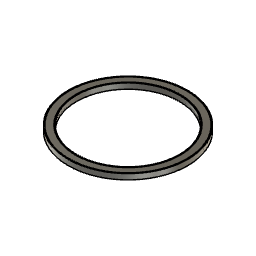
silicon_gasket_mold (Autodesk Fusion 360 design; units mm, degrees)
Autodesk Fusion 360 part; units mm, degrees
sketch "Sketch1" plane through (0, 0, 0) normal (0, 0, 1) x (1, 0, 0)
  circle A0 centre (0, 0) radius 91.5
  circle A1 centre (0, 0) radius 93
  circle A2 centre (0, 0) radius 81.5
  circle A3 centre (0, 0) radius 80
  line L0 (0, 0) -> (-81.5, 0) construction
  line L1 (-91.5, 0, 0) -> (-91.5, 0, 2.6785)
  line L2 (-81.5, 0, 0) -> (-91.5, 0, 2.6785)
  line L3 (-91.5, 0) -> (-81.5, 0)
  dimension "d1" = 183
  dimension "d2" = 1.5
  dimension "d3" = 163
  dimension "d4" = -1.5
  constraint coincident A0.centre A1.centre
  constraint concentric A0 A2
  constraint coincident A2 L0.end
  constraint horizontal L0
  constraint coincident A0 L3.start
  measures "d1" diameter of A0
  measures "d3" diameter of A2
extrude "Extrude1" add sketch "Sketch1" against normal blind 1.5 contours A0 | A1 | A2 makes body 1
extrude "Extrude2" add sketch "Sketch1" along normal blind 7 bodies 1
revolve "Revolve1" add sketch "Sketch1" angle 360 about axis through (0, 0, 1.75) along (0, 0, 1) contours L1 L2 L3 in plane through (0, 0, 0) normal (0, 1, 0) bodies 1
sketch "Sketch2" plane through (0, 0, 0) normal (0, 1, 0) x (1, 0, 0)
  line L0 (81.5, 0) -> (-81.5, 0)
  line L1 (91.5, -2.6785) -> (-91.5, -2.6785)
  line L2 (-91.5, -2.6785) -> (-81.5, 0)
  line L3 (-81.5, -7) -> (81.5, -7)
  line L4 (91.5, -7) -> (-91.5, -7)
  line L5 (-81.5, 0) -> (-81.5, -7)
  line L6 (-81.5, -7) -> (-91.5, -7)
  line L7 (-91.5, -2.6785) -> (-91.5, -7)
  constraint coincident L1.end L2.start
  constraint coincident L0.end L2.end
  constraint coincident L3.start L5.end
  constraint coincident L4.end L6.end
revolve "Revolve2" add sketch "Sketch2" angle 360 about axis through (0, 0, 1.75) along (0, 0, 1) separate body makes body 2
